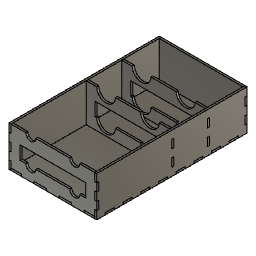
Verkefni_2_vinfloskustandur (Autodesk Fusion 360 design; units mm, degrees)
Autodesk Fusion 360 part; units mm, degrees
sketch "vinstri hlid sketch" plane through (0, 0, 0) normal (1, 0, 0) x (0, 1, 0)
  line L0 (0, 0) -> (300, 0)
  line L1 (300, 0) -> (300, 80)
  line L2 (300, 80) -> (0, 80)
  line L3 (0, 80) -> (0, 0)
  dimension "d11" = 300
  dimension "d12" = 80
  constraint perpendicular L0 L1
  constraint parallel L0 L2
  constraint parallel L1 L3
  constraint horizontal L0
  constraint coincident L0.start L3.end
  measures "d11" distance of L0.start L0.end
  measures "d12" distance of L0.start L2.end
extrude "Extrude1" add sketch "vinstri hlid sketch" along normal blind 4 makes body 1
sketch "fingur hlid sketch" plane through (0, 0, 0) normal (0, 0, 1) x (1, 0, 0)
  line L0 (0, 17.6471) -> (4, 17.6471)
  line L1 (4, 17.6471) -> (4, 35.2941)
  line L2 (4, 35.2941) -> (0, 35.2941)
  line L3 (0, 35.2941) -> (0, 17.6471)
  dimension "d15" = 17.6471
  dimension "d16" = 17.6471
  constraint horizontal L0
  constraint vertical L1
  constraint horizontal L2
  constraint vertical L3
  measures "d15" distance of L0.end L1.end
  measures "d16" distance of origin L0
extrude "Extrude2" cut sketch "fingur hlid sketch" along normal blind 4 bodies 1
pattern_linear "R-Pattern1" count 8 spacing 35.2941 along (0, 1, 0) of "Extrude2"
sketch "Botn sketch" plane through (0, 0, 0) normal (0, 0, 1) x (1, 0, 0)
  line L0 (0, 0) -> (0, 300)
  line L1 (0, 300) -> (175, 300)
  line L2 (175, 300) -> (175, 0)
  line L3 (175, 0) -> (0, 0)
  dimension "d23" = 300
  dimension "d24" = 175
  constraint perpendicular L0 L1
  constraint parallel L0 L2
  constraint parallel L1 L3
  constraint vertical L0
  constraint coincident L0.start L3.end
  measures "d23" distance of L0.start L0.end
  measures "d24" distance of L0.start L2.end
extrude "Extrude3" add sketch "Botn sketch" along normal blind 4 separate body makes body 2
combine "Combine1" operation cut target body 2 tool bodies 1 keep tools
sketch "Sketch4" plane through (0, 0, 0) normal (0, 1, 0) x (1, 0, 0)
  line L0 (0, -16) -> (4, -16)
  line L1 (4, -16) -> (4, -32)
  line L2 (4, -32) -> (0, -32)
  line L3 (0, -32) -> (0, -16)
  dimension "d27" = 16
  dimension "d28" = 16
  constraint horizontal L0
  constraint vertical L1
  constraint horizontal L2
  constraint vertical L3
  measures "d27" distance of L0.start L2.end
  measures "d28" distance of L0 origin
extrude "Extrude4" cut sketch "Sketch4" along normal blind 4 bodies 1
pattern_linear "R-Pattern2" count 2 spacing 32 along (0, 0, 1) of "Extrude4"
sketch "fingur botn sketch" plane through (0, 0, 0) normal (0, 1, 0) x (1, 0, 0)
  line L0 (25, 0) -> (50, 0)
  line L1 (50, 0) -> (50, -4)
  line L2 (50, -4) -> (25, -4)
  line L3 (25, -4) -> (25, 0)
  dimension "d35" = 25
  dimension "d36" = 25
  constraint horizontal L0
  constraint vertical L1
  constraint horizontal L2
  constraint vertical L3
  measures "d35" distance of L0.start L0.end
  measures "d36" distance of L3 origin
extrude "Extrude5" cut sketch "fingur botn sketch" along normal blind 4 bodies 2
pattern_linear "R-Pattern3" count 3 spacing 50 along (1, 0, 0) of "Extrude5"
extrude "Extrude6" add 1 faces at (0, 152.9412, 54.6667) along direction (-1, 0, 0) blind 4 from surface at -175 separate body on bodies 1 makes body 3
combine "Combine2" operation cut target body 2 tool bodies 3 keep tools
combine "Combine4" operation cut target body 1 tool bodies 2 keep tools
combine "Combine5" operation cut target body 2 tool bodies 3 keep tools
sketch "AFtur hluti sketch" plane through (0, 0, 0) normal (0, 1, 0) x (1, 0, 0)
  line L0 (0, 0) -> (175, 0)
  line L1 (175, 0) -> (175, -80)
  line L2 (175, -80) -> (0, -80)
  line L3 (0, -80) -> (0, 0)
  dimension "d65" = 175
  dimension "d66" = 80
  constraint perpendicular L0 L1
  constraint parallel L0 L2
  constraint parallel L1 L3
  constraint horizontal L0
  constraint coincident L0.start L3.end
  measures "d65" distance of L0.start L0.end
  measures "d66" distance of L0.start L2.end
extrude "Extrude9" add sketch "AFtur hluti sketch" along normal blind 4 separate body makes body 4
combine "Combine7" operation cut target body 4 tool bodies 1 3 2 keep tools
move_body "Move2" bodies 4 to x (1, 0, 0) y (0, 1, 0) z (0, 0, 1) at (0, 296, 0)
combine "Combine8" operation cut target body 1 tool bodies 4 keep tools
combine "Combine9" operation cut target body 2 tool bodies 4 keep tools
combine "Combine10" operation cut target body 3 tool bodies 4 keep tools
sketch "Milli haldari sketch" plane through (0, 0, 0) normal (0, 1, 0) x (1, 0, 0)
  line L0 (0, 0) -> (175, 0)
  line L1 (175, 0) -> (175, -80)
  line L2 (175, -80) -> (0, -80)
  line L3 (0, -80) -> (0, 0)
  line L4 (0, -80) -> (43.75, -80)
  circle A0 centre (43.75, -80) radius 18.625
  line L5 (0, -80) -> (131.25, -80)
  circle A1 centre (131.25, -80) radius 18.625
  line L6 (0, 0) -> (0, -26.6667)
  circle A2 centre (43.75, -26.6667) radius 18.625
  circle A3 centre (131.25, -26.6667) radius 18.625
  line L7 (21.875, -26.6667) -> (21.875, -53.3333)
  line L8 (21.875, -53.3333) -> (153.125, -53.3333)
  line L9 (153.125, -53.3333) -> (153.125, -26.6667)
  line L10 (21.875, -26.6667) -> (153.125, -26.6667)
  dimension "d80" = 175
  dimension "d81" = 80
  dimension "d82" = 43.75
  dimension "d83" = 37.25
  dimension "d84" = 131.25
  dimension "d85" = 37.25
  dimension "d88" = 26.6667
  dimension "d89" = 43.75
  dimension "d90" = 37.25
  dimension "d91" = 131.25
  dimension "d92" = 37.25
  dimension "d95" = 21.875
  dimension "d96" = 26.6667
  dimension "d97" = 131.25
  dimension "d98" = 26.6667
  constraint perpendicular L0 L1
  constraint parallel L0 L2
  constraint parallel L1 L3
  constraint horizontal L0
  constraint coincident L0.start L3.end
  constraint perpendicular L3 L4
  constraint coincident L4.end A0.centre
  constraint perpendicular L3 L5
  constraint coincident L5.end A1.centre
  constraint coincident L3 L6.end
  constraint perpendicular L7 L8
  constraint perpendicular L9 L10
  measures "d80" distance of L0.start L0.end
  measures "d81" distance of L0.start L2.end
  measures "d82" distance of L2.end L4.end
  measures "d83" diameter of A0
  measures "d84" distance of L2.end L5.end
  measures "d85" diameter of A1
  measures "d88" distance of L0.start L6.end
  measures "d89" distance of L6.end A2.centre
  measures "d90" diameter of A2
  measures "d91" distance of L6.end A3.centre
  measures "d92" diameter of A3
  measures "d95" distance of L6.end L7.start
  measures "d96" distance of L7.start L7.end
  measures "d97" distance of L7.end L8.end
  measures "d98" distance of L8.end L9.end
extrude "Extrude10" add sketch "Milli haldari sketch" along normal blind 4 separate body contours L0 L1 L2 L3 L4 A0 L5 A1 L6 makes body 5
combine "Combine11" operation cut target body 5 tool bodies 1 3 2 keep tools
sketch "Sketch13" plane through (0, 4, 0) normal (0, 1, 0) x (-1, 0, 0)
  line L0 (-21.875, 26.6667) -> (-25.125, 26.6667)
  arc A0 (-62.375, 26.6667) -> (-25.125, 26.6667) centre (-43.75, 26.6667) ccw
  arc A1 (-149.875, 26.6667) -> (-112.625, 26.6667) centre (-131.25, 26.6667) ccw
  line L1 (-171, 4) -> (-150, 4)
  line L2 (-150, 4) -> (-150, 0)
  line L3 (-150, 0) -> (-125, 0)
  line L4 (-125, 0) -> (-125, 4)
  line L5 (-125, 4) -> (-100, 4)
  line L6 (-100, 4) -> (-100, 0)
  line L7 (-100, 0) -> (-75, 0)
  line L8 (-75, 0) -> (-75, 4)
  line L9 (-75, 4) -> (-50, 4)
  line L10 (-50, 4) -> (-50, 0)
  line L11 (-50, 0) -> (-25, 0)
  line L12 (-25, 0) -> (-25, 4)
  line L13 (-25, 4) -> (-4, 4)
  line L14 (-4, 4) -> (-4, 16)
  line L15 (-4, 16) -> (0, 16)
  line L16 (0, 16) -> (0, 32)
  line L17 (0, 32) -> (-4, 32)
  line L18 (-4, 32) -> (-4, 48)
  line L19 (-4, 48) -> (0, 48)
  line L20 (0, 48) -> (0, 64)
  line L21 (0, 64) -> (-4, 64)
  line L22 (-4, 64) -> (-4, 80)
  line L23 (-4, 80) -> (-25.125, 80)
  arc A2 (-62.375, 80) -> (-25.125, 80) centre (-43.75, 80) ccw
  line L24 (-62.375, 80) -> (-112.625, 80)
  arc A3 (-149.875, 80) -> (-112.625, 80) centre (-131.25, 80) ccw
  line L25 (-149.875, 80) -> (-171, 80)
  line L26 (-171, 80) -> (-171, 64)
  line L27 (-171, 64) -> (-175, 64)
  line L28 (-175, 64) -> (-175, 48)
  line L29 (-175, 48) -> (-171, 48)
  line L30 (-171, 48) -> (-171, 32)
  line L31 (-171, 32) -> (-175, 32)
  line L32 (-175, 32) -> (-175, 16)
  line L33 (-175, 16) -> (-171, 16)
  line L34 (-171, 16) -> (-171, 4)
  line L35 (-21.875, 53.3333) -> (-21.875, 26.6667)
  line L36 (-149.875, 26.6667) -> (-153.125, 26.6667)
  line L37 (-153.125, 26.6667) -> (-153.125, 53.3333)
  line L38 (-153.125, 53.3333) -> (-21.875, 53.3333)
  line L39 (-62.375, 26.6667) -> (-112.625, 26.6667)
extrude "Extrude11" add 1 faces at (91.6667, 4, 19.1111) along direction (0, -1, 0) blind 4 from surface at -221 separate body on bodies 5 makes body 6
move_body "Move3" bodies 5 to x (1, 0, 0) y (0, 1, 0) z (0, 0, 1) at (0, 150, 0)
combine "Combine12" operation cut target body 3 tool bodies 6 5 keep tools
combine "Combine13" operation cut target body 1 tool bodies 6 5 keep tools
combine "Combine14" operation cut target body 2 tool bodies 6 5 keep tools
sketch "Sketch14" plane through (0, 0, 0) normal (0, 1, 0) x (1, 0, 0)
  line L0 (0, 0) -> (175, 0)
  line L1 (175, 0) -> (175, -80)
  line L2 (175, -80) -> (0, -80)
  line L3 (0, -80) -> (0, 0)
  line L4 (0, -80) -> (43.75, -80)
  line L5 (0, -80) -> (131.25, -80)
  circle A0 centre (43.75, -80) radius 10
  circle A1 centre (131.25, -80) radius 10
  line L6 (0, 0) -> (0, -26.6667)
  circle A2 centre (43.75, -26.6667) radius 10
  circle A3 centre (131.25, -26.6667) radius 10
  line L7 (21.875, -26.6667) -> (21.875, -53.3333)
  line L8 (21.875, -53.3333) -> (153.125, -53.3333)
  line L9 (153.125, -53.3333) -> (153.125, -26.6667)
  line L10 (21.875, -26.6667) -> (153.125, -26.6667)
  dimension "d104" = 175
  dimension "d105" = 80
  dimension "d106" = 43.75
  dimension "d107" = 131.25
  dimension "d108" = 20
  dimension "d109" = 20
  dimension "d110" = 26.6667
  dimension "d111" = 43.75
  dimension "d112" = 131.25
  dimension "d113" = 20
  dimension "d114" = 20
  dimension "d115" = 21.875
  dimension "d116" = 26.6667
  dimension "d117" = 131.25
  dimension "d118" = 26.6667
  dimension "d119" = 131.25
  constraint perpendicular L0 L1
  constraint parallel L0 L2
  constraint parallel L1 L3
  constraint horizontal L0
  constraint coincident L0.start L3.end
  constraint coincident L2 L4.end
  constraint perpendicular L3 L5
  constraint coincident L4.end A0.centre
  constraint coincident L5.end A1.centre
  constraint coincident L3 L6.end
  constraint perpendicular L6 L8
  measures "d104" distance of L0.start L0.end
  measures "d105" distance of L0.start L2.end
  measures "d106" distance of L2.end L4.end
  measures "d107" distance of L2.end L5.end
  measures "d108" diameter of A0
  measures "d109" diameter of A1
  measures "d110" distance of L0.start L6.end
  measures "d111" distance of L6.end A2.centre
  measures "d112" distance of L6.end A3.centre
  measures "d113" diameter of A2
  measures "d114" diameter of A3
  measures "d115" distance of L6.end L7.start
  measures "d116" distance of L7.start L7.end
  measures "d117" distance of L7.end L8.end
  measures "d118" distance of L8.end L9.end
  measures "d119" distance of L7.start L9.end
extrude "Extrude12" add sketch "Sketch14" along normal blind 4 separate body contours L0 L1 L2 L3 L4 L5 A0 A1 L6 makes body 7
combine "Combine15" operation cut target body 7 tool bodies 1 3 2 keep tools
equation "lengd = 300 mm" comment "Heildar lengd"
equation "breydd = 175 mm" comment "Heildar breydd"
equation "haed = 80 mm" comment "Heildar hæð"
equation "þykkt = 4 mm" comment "Þykkt efnis"
equation "fjoldi_f_h = 2" comment "Fjoldi fingra á hæðinni"
equation "fjoldi_f_b = 3" comment "Fjöldi fingra á breydd"
equation "fjoldi_f_l = 8" comment "Fjöldi fingra á lengd"
equation "lengd_fingra = lengd / ( ( fjoldi_f_l * 2 ) + 1 )" comment "lengd fingrana"
equation "breydd_fingra = breydd / ( ( fjoldi_f_b * 2 ) + 1 )" comment "Dýpt fingrana"
equation "haed_fingra = haed / ( ( fjoldi_f_h * 2 ) + 1 )" comment "Hæð fingra"
equation "d11 = lengd"
equation "d12 = haed"
equation "d13 = þykkt"
equation "d15 = lengd_fingra"
equation "d16 = lengd_fingra"
equation "d17 = þykkt"
equation "d19 = fjoldi_f_l"
equation "d21 = lengd - ( lengd_fingra * 3 )"
equation "d23 = lengd"
equation "d24 = breydd"
equation "d25 = þykkt"
equation "d27 = haed_fingra"
equation "d28 = haed_fingra"
equation "d29 = þykkt"
equation "d31 = fjoldi_f_h"
equation "d33 = -haed + haed_fingra * 3"
equation "d35 = breydd_fingra"
equation "d36 = breydd_fingra"
equation "d37 = þykkt"
equation "d39 = fjoldi_f_b"
equation "d41 = -breydd + breydd_fingra * 3"
equation "d43 = -breydd"
equation "d44 = þykkt"
equation "R_aftan = 37.25 mm" comment "Rafdíus hringsins fyrir flösku enda"
equation "R_framan = 20 mm" comment "Radíus hringsins að framan"
equation "d65 = breydd"
equation "d66 = haed"
equation "d67 = þykkt"
equation "d80 = breydd"
equation "d81 = haed"
equation "d82 = breydd / 4"
equation "d83 = R_aftan"
equation "d84 = ( breydd / 4 ) * 3"
equation "d85 = R_aftan"
equation "d88 = haed / 3"
equation "d89 = breydd / 4"
equation "d90 = R_aftan"
equation "d91 = ( breydd / 4 ) * 3"
equation "d92 = R_aftan"
equation "d95 = breydd / 8"
equation "d96 = haed / 3"
equation "d97 = ( breydd / 8 ) * 6"
equation "d98 = haed / 3"
equation "d99 = þykkt"
equation "d101 = -( lengd / 4 ) * 1"
equation "d102 = -þykkt"
equation "d104 = breydd"
equation "d105 = haed"
equation "d106 = breydd / 4"
equation "d107 = ( breydd / 4 ) * 3"
equation "d108 = R_framan"
equation "d109 = R_framan"
equation "d110 = haed / 3"
equation "d111 = breydd / 4"
equation "d112 = ( breydd / 4 ) * 3"
equation "d113 = R_framan"
equation "d114 = R_framan"
equation "d115 = breydd / 8"
equation "d116 = haed / 3"
equation "d117 = ( breydd / 8 ) * 6"
equation "d118 = haed / 3"
equation "d119 = ( breydd / 8 ) * 6"
equation "d120 = þykkt"
named bodies: "Vinstri lengd", "Botn", "hægri lengd", "Aftur hluti", "Fremri haldari", "Aftrari haldari", "Framhlið"
